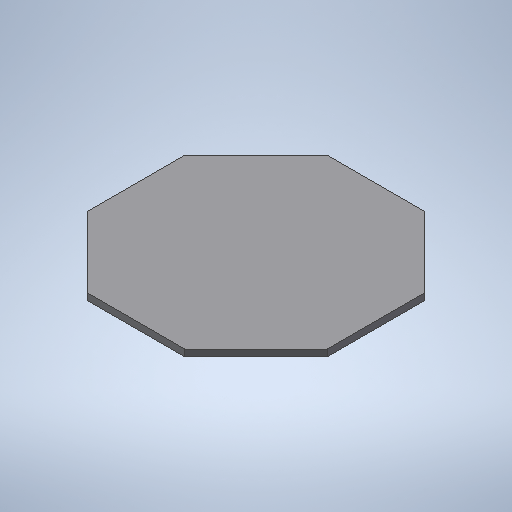
# Autodesk Inventor part: 上板
Saved by Autodesk Inventor 2025.2 (Build 292293000, 293)
## iProperties
Created: 2026-03-19
Part Number: 上板
Material: 常规
Document SubType Name: Modeling
Designer: BO‘S_SLAVE
Density: 1 g/cm^3
Appearance: 默认
Author: BO‘S_SLAVE
Autodesk Inventor part; units mm, degrees
ref_plane "YZ Plane" through (0, 0, 0) normal (1, 0, 0) x (0, 1, 0)
ref_plane "XZ Plane" through (0, 0, 0) normal (0, 1, 0) x (-1, 0, 0)
ref_plane "XY Plane" through (0, 0, 0) normal (0, 0, 1) x (1, 0, 0)
sketch "草图1" plane through (0, 0, 0) normal (0, 1, 0) x (-1, 0, 0)
  line L0 (25.1023, 25.1023) -> (-25.1023, 25.1023)
  line L1 (-25.1023, 25.1023) -> (-25.1023, -25.1023)
  line L2 (-25.1023, -25.1023) -> (25.1023, -25.1023)
  line L3 (25.1023, -25.1023) -> (25.1023, 25.1023)
  line L4 (25.1023, 25.1023) -> (-25.1023, -25.1023)
  line L5 (25.1023, -25.1023) -> (-25.1023, 25.1023)
  line L6 (-14.4957, 35.7089) -> (-35.7089, 14.4957)
  line L7 (-35.7089, -14.4957) -> (-14.4957, -35.7089)
  line L8 (14.4957, -35.7089) -> (35.7089, -14.4957)
  line L9 (35.7089, 14.4957) -> (14.4957, 35.7089)
  line L10 (14.4957, 35.7089) -> (-14.4957, 35.7089)
  line L11 (35.7089, 14.4957) -> (35.7089, -14.4957)
  line L12 (14.4957, -35.7089) -> (-14.4957, -35.7089)
  line L13 (-35.7089, -14.4957) -> (-35.7089, 14.4957)
  circle A0 centre (16.9706, 16.9706) radius 1.65
  circle A1 centre (14.8492, 30.4056) radius 1.65
  circle A2 centre (30.4056, 14.8492) radius 1.65
  point P0 (0, 0)
  point P1 (0, 0)
  point P2 (-25.1023, -25.1023)
  point P3 (25.1023, 25.1023)
  dimension "d0" = 71
  dimension "d1" = 30
  dimension "d2" = 45
  dimension "d5" = 360
  constraints: 28 end point, 6 perpendicular, 3 centre point, 2 midpoint, 2 parallel, 1 coincident, 1 horizontal, 17 other
  measures "d0" distance of L2.end L0.end
  measures "d1" distance of L6.start L6.end
  measures "d2" angle of L6 L1
extrude "拉伸1" add sketch "草图1" along normal blind 2 contours L4 A0 L5 L0 | L9 L11 L8 L3 | L3 L5 L4 A0 | L0 L6 L10 L9 | L5 L4 L1 | L1 L7 L13 L6 | L8 L12 L7 L2 | L2 L4 L5 | A0 L4 | L4 A0 | A1 | A2
